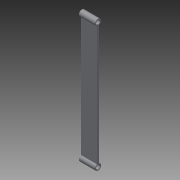
# Autodesk Inventor part: aimingcontrol
Saved by Autodesk Inventor 2016 (Build 200138000, 138)
## iProperties
Created: 2016-01-30
Part Number: aimingcontrol
Material: Generic
Document SubType Name: Modeling
Designer: zachary
Density: 1 g/cm^3
Appearance: Default
Mass: 18.6686 g
Surface Area: 143.506 cm^2
Volume: 18.6686 cm^3
Author: zachary
Autodesk Inventor part; units mm, degrees
ref_plane "YZ Plane" through (0, 0, 0) normal (1, 0, 0) x (0, 1, 0)
ref_plane "XZ Plane" through (0, 0, 0) normal (0, 1, 0) x (-1, 0, 0)
ref_plane "XY Plane" through (0, 0, 0) normal (0, 0, 1) x (1, 0, 0)
sketch "Sketch1" plane through (0, 0, 0) normal (1, 0, 0) x (0, 1, 0)
  line L0 (204.9689, 1.6371) -> (-1.9508, 1.6371)
  line L1 (-1.9508, -1.5379) -> (204.9689, -1.5379)
  circle A0 centre (-6.441, 0.0496) radius 3.175
  circle A1 centre (209.459, 0.0496) radius 3.175
  arc A2 (-1.9508, 1.6371) -> (-1.9508, -1.5379) centre (-6.441, 0.0496) ccw
  arc A3 (204.9689, -1.5379) -> (204.9689, 1.6371) centre (209.459, 0.0496) ccw
  point P0 (0, 0)
  dimension "d0" = 3.175
  dimension "d2" = 6.35
  dimension "d3" = 6.35
  dimension "d4" = 1.5875
  dimension "d5" = 1.5875
  dimension "d8" = 215.9
  constraints: 4 centre point, 4 end point, 4 point on circle, 2 coincident, 1 horizontal, 1 parallel
  measures "d0" distance between parallel lines of L0 L1
  measures "d2" diameter of A1
  measures "d3" diameter of A0
  measures "d4" radial gap between concentric circles of A1 A3
  measures "d5" radial gap between concentric circles of A0 A2
  measures "d8" distance of A1.centre A0.centre
extrude "Extrusion1" add sketch "Sketch1" along normal blind 25.4
body "Solid1"
